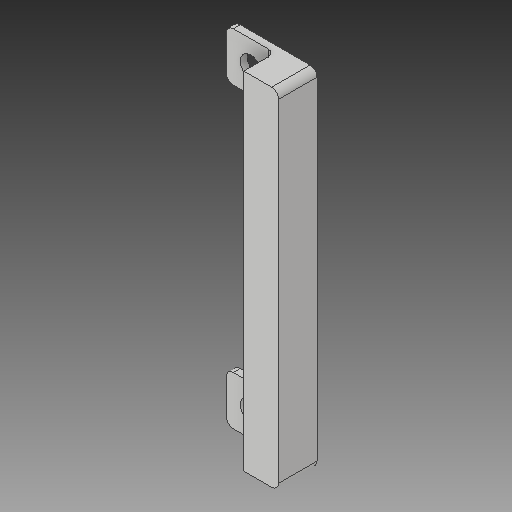
# Autodesk Inventor part: BaseSyringeRackWall
Saved by Autodesk Inventor 2018 (Build 220112000, 112)
## iProperties
Created: 2018-05-20
Part Number: BaseSyringeRackWall
Material: Generic
Document SubType Name: Modeling
Designer: reide
Density: 1 g/cm^3
Appearance: Default
Author: reide
Autodesk Inventor part; units mm, degrees
ref_plane "YZ Plane" through (0, 0, 0) normal (1, 0, 0) x (0, 1, 0)
sketch "Sketch1" plane through (0, 0, 0) normal (0, 0, 1) x (1, 0, 0)
  arc A0 (-46.3358, 172.7675) -> (-47.3358, 171.7675) centre (-46.3358, 171.7675) ccw projected
  line L0 (-47.3358, 135.0985) -> (-47.3358, 171.7675) projected
  line L1 (-47.3358, 135.0985) -> (-45.6213, 135.0985) projected
  line L2 (-45.6213, 135.0985) -> (-45.6213, 137.2488) projected
  line L3 (-45.6213, 137.2488) -> (-39.2713, 137.2488) projected
  line L4 (-39.2713, 137.2488) -> (-39.2713, 135.0985) projected
  line L5 (-39.2713, 135.0985) -> (-37.5568, 135.0985) projected
  line L6 (-37.5568, 171.7675) -> (-37.5568, 135.0985) projected
  arc A1 (-37.5568, 171.7675) -> (-38.5568, 172.7675) centre (-38.5568, 171.7675) ccw projected
  line L7 (-38.5568, 172.7675) -> (-46.3358, 172.7675) projected
  line L8 (-39.2713, 143.7065) -> (-39.2713, 141.5562) projected
  line L9 (-39.2713, 141.5562) -> (-45.6213, 141.5562) projected
  line L10 (-45.6213, 141.5562) -> (-45.6213, 143.7065) projected
  line L11 (-45.6213, 143.7065) -> (-39.2713, 143.7065) projected
  line L12 (-39.2713, 150.1642) -> (-39.2713, 148.0139) projected
  line L13 (-39.2713, 148.0139) -> (-45.6213, 148.0139) projected
  line L14 (-45.6213, 148.0139) -> (-45.6213, 150.1642) projected
  line L15 (-45.6213, 150.1642) -> (-39.2713, 150.1642) projected
  line L16 (-39.2713, 156.622) -> (-39.2713, 154.4717) projected
  line L17 (-39.2713, 154.4717) -> (-45.6213, 154.4717) projected
  line L18 (-45.6213, 154.4717) -> (-45.6213, 156.622) projected
  line L19 (-45.6213, 156.622) -> (-39.2713, 156.622) projected
  line L20 (-39.2713, 163.0797) -> (-39.2713, 160.9294) projected
  line L21 (-39.2713, 160.9294) -> (-45.6213, 160.9294) projected
  line L22 (-45.6213, 160.9294) -> (-45.6213, 163.0797) projected
  line L23 (-45.6213, 163.0797) -> (-39.2713, 163.0797) projected
  line L24 (-39.2713, 169.5375) -> (-39.2713, 167.3871) projected
  line L25 (-39.2713, 167.3871) -> (-45.6213, 167.3871) projected
  line L26 (-45.6213, 167.3871) -> (-45.6213, 169.5375) projected
  line L27 (-45.6213, 169.5375) -> (-39.2713, 169.5375) projected
  line L28 (-39.2713, 172.7663) -> (-39.2713, 170.616) projected
  line L29 (-39.2713, 170.616) -> (-45.6213, 170.616) projected
  line L30 (-45.6213, 170.616) -> (-45.6213, 172.7663) projected
  line L31 (-45.6213, 172.7663) -> (-39.2713, 172.7663) projected
  line L32 (-39.2713, 166.3086) -> (-39.2713, 164.1583) projected
  line L33 (-39.2713, 164.1583) -> (-45.6213, 164.1583) projected
  line L34 (-45.6213, 164.1583) -> (-45.6213, 166.3086) projected
  line L35 (-45.6213, 166.3086) -> (-39.2713, 166.3086) projected
  line L36 (-39.2713, 159.8508) -> (-39.2713, 157.7005) projected
  line L37 (-39.2713, 157.7005) -> (-45.6213, 157.7005) projected
  line L38 (-45.6213, 157.7005) -> (-45.6213, 159.8508) projected
  line L39 (-45.6213, 159.8508) -> (-39.2713, 159.8508) projected
  line L40 (-39.2713, 153.3931) -> (-39.2713, 151.2428) projected
  line L41 (-39.2713, 151.2428) -> (-45.6213, 151.2428) projected
  line L42 (-45.6213, 151.2428) -> (-45.6213, 153.3931) projected
  line L43 (-45.6213, 153.3931) -> (-39.2713, 153.3931) projected
  line L44 (-39.2713, 146.9354) -> (-39.2713, 144.7851) projected
  line L45 (-39.2713, 144.7851) -> (-45.6213, 144.7851) projected
  line L46 (-45.6213, 144.7851) -> (-45.6213, 146.9354) projected
  line L47 (-45.6213, 146.9354) -> (-39.2713, 146.9354) projected
  line L48 (-39.2713, 140.4776) -> (-39.2713, 138.3273) projected
  line L49 (-39.2713, 138.3273) -> (-45.6213, 138.3273) projected
  line L50 (-45.6213, 138.3273) -> (-45.6213, 140.4776) projected
  line L51 (-45.6213, 140.4776) -> (-39.2713, 140.4776) projected
  line L52 (-32.1913, 173.114) -> (-36.2913, 173.114) projected
  arc A2 (-36.2913, 173.114) -> (-37.2913, 172.114) centre (-36.2913, 172.114) ccw projected
  line L53 (-37.2913, 172.114) -> (-37.2913, 124.114) projected
  arc A3 (-37.2913, 124.114) -> (-36.2913, 123.114) centre (-36.2913, 124.114) ccw projected
  line L54 (-36.2913, 123.114) -> (-30.1913, 123.114) projected
  arc A4 (-30.1913, 123.114) -> (-29.1913, 124.114) centre (-30.1913, 124.114) ccw projected
  line L55 (-29.1913, 124.114) -> (-29.1913, 133.114) projected
  line L56 (-29.1913, 133.114) -> (-32.1913, 133.114) projected
  arc A5 (-34.1913, 135.114) -> (-32.1913, 133.114) centre (-32.1913, 135.114) ccw projected
  line L57 (-34.1913, 135.114) -> (-34.1913, 171.114) projected
  arc A6 (-32.1913, 173.114) -> (-34.1913, 171.114) centre (-32.1913, 171.114) ccw projected
  line L58 (-32.1913, 173.114) -> (-36.2913, 173.114) projected
  line L59 (-47.3358, 172.7663) -> (-47.8358, 172.7663)
  line L60 (-47.8358, 172.7663) -> (-47.8358, 123.114)
  line L61 (-47.8358, 123.114) -> (-52.8358, 123.114)
  line L62 (-52.8358, 123.114) -> (-47.8358, 123.114)
  line L63 (-47.8358, 123.114) -> (-47.8358, 172.7663)
  line L64 (-47.8358, 172.7663) -> (-52.8358, 172.7663)
  line L65 (-52.8358, 172.7663) -> (-52.8358, 123.114)
  point P0 (0, 0)
  dimension "d0" = 0.5
  dimension "d1" = 5
  constraints: 14 end point, 2 horizontal, 2 parallel, 2 perpendicular, 2 point on line
  measures "d0" distance of L59.start L59.end
  measures "d1" distance of L60.end L61.end
ref_plane "Work Plane1" through (-47.3358, 135.0985, 5.5) normal (0, 0, 1) x (1, 0, 0)
extrude "Extrusion1" add sketch "Sketch1" along normal up to surface (5.5 mm away) contours L60 L61 L65 L64
ref_plane "Work Plane2" through (-21.046, 260.6747, 1) normal (0, 0, 1) x (1, 0, 0)
sketch "Sketch2" plane through (0, 0, 0) normal (0, 0, -1) x (-1, 0, 0)
  line L0 (21.046, 191.8247) -> (21.046, 196.1747) projected
  line L1 (20.046, 197.1747) -> (14.696, 197.1747) projected
  line L2 (-10.466, 190.8247) -> (20.046, 190.8247) projected
  line L3 (47.8358, 172.7663) -> (52.8358, 172.7663) projected
  line L4 (52.8358, 172.7663) -> (59.8358, 172.7663)
  line L5 (59.8358, 172.7663) -> (59.8358, 165.7663)
  line L6 (59.8358, 165.7663) -> (52.8358, 165.7663)
  line L7 (52.8358, 165.7663) -> (52.8358, 172.7663)
  circle A0 centre (56.3358, 169.2663) radius 1.5
  line L8 (52.8358, 172.7663) -> (52.8358, 123.114) projected
  line L9 (52.8358, 147.9401) -> (59.0702, 147.9401)
  line L10 (47.8358, 123.114) -> (52.8358, 123.114)
  line L11 (52.8358, 123.114) -> (59.8358, 123.114)
  line L12 (59.8358, 123.114) -> (59.8358, 130.114)
  line L13 (59.8358, 130.114) -> (52.8358, 130.114)
  line L14 (52.8358, 130.114) -> (52.8358, 123.114)
  circle A1 centre (56.3358, 126.614) radius 1.5
  line L15 (52.8358, 123.114) -> (52.8358, 172.7663)
  point P0 (0, 0)
  point P1 (59.8358, 169.2663)
  point P2 (59.8358, 126.614)
  dimension "d4" = 7
  dimension "d5" = 7
  dimension "d6" = 3
  constraints: 22 end point, 8 symmetric about line, 2 centre point, 2 horizontal, 2 midpoint, 2 parallel, 1 perpendicular, 1 other
  measures "d4" distance of L5.end L6.end
  measures "d5" distance of L4.end L5.end
  measures "d6" diameter of A0
extrude "Extrusion2" add sketch "Sketch2" against normal up to surface (1 mm away)
fillet "Fillet1" radius 1 4 edges at (-59.8358, 172.7663, 0.5) (-59.8358, 165.7663, 0.5) (-59.8358, 123.114, 0.5) (-59.8358, 130.114, 0.5)
fillet "Fillet2" radius 1 2 edges at (-52.8358, 169.2663, 1) (-52.8358, 126.614, 1)
fillet "Fillet3" radius 1 2 edges at (-47.8358, 172.7663, 2.75) (-47.8358, 123.114, 2.75)
body "Solid1"
